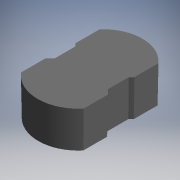
# Autodesk Inventor part: LZ80_Gehaeuse_Parallelform
Saved by Autodesk Inventor 2021 (Build 250183000, 183)
## iProperties
Part Number: LZ80_Gehaeuse_Parallelform
Material: Generic
Catalog Web Link: www.cadenas.de
Description: LZ80 Gehaeuse Parallelform-Bauteil LZ80
Vendor: ROSEKRIEGER
Document SubType Name: Modeling
Designer: partserver
Manufacturer: ROSEKRIEGER
Mass: 1239.51 g
Surface Area: 731.392 cm^2
Volume: 1239.51 cm^3
Density: 1 g/cm^3
Appearance: PSOLRGB-128-128-128
Category: PARTsolutions
Company: ROSEKRIEGER
PSOL_IDENT_0: {$CADENAS_DATA\23d-libs\rose_krieger\linearkomponenten\pool_lineartechnik\_hubsaeule_zyliinder\elekt
PSOL_IDENT_1: rozylinder\elekzyl_lz80\lz80_gehaeuse_parallelform.prj},203 {VTYP=3D},{NB=LZ80_Gehaeuse_Parallelform
PSOL_IDENT_2: },{LINA=LZ80_Gehaeuse_Parallelform},{NN=LZ80 Gehaeuse Parallelform},{DATE=02.12.2020 11:16:40},{GEOM
PSOL_IDENT_3: DATE=12.12.2006},{VERSION=},{LINEID=10},{WBVAR=},{WBNUMERIC=}  {NB=LZ80_Gehaeuse_Parallelform},{LINA=
PSOL_IDENT_4: LZ80_Gehaeuse_Parallelform},{KT=DUMMY},{IDNR=},{ARTIKEL=LZ80_Gehaeuse_Parallelform},{DECKELBR1=107.3
PSOL_IDENT_5: 10},{DECKELBR2=114.310},{DECKELBR3=97.310},{KONTRA1=71.450},{KONTRA2=74.100},{ABKONTRA2=25.250},{ABK
PSOL_IDENT_6: ONTRA1=25.240},{ACHSAB=95.760},{HOEHE=67.000},{ABBEFBO1=56.500},{NUTTIEF=0.100},{NUTBREIT=12.000}
NB: LZ80_Gehaeuse_Parallelform
NN: LZ80 Gehaeuse Parallelform
NT: Bauteil LZ80
NBSYN: $ARTIKEL.
LINA: LZ80_Gehaeuse_Parallelform
CATALOG: RK Rose+Krieger
ARTIKEL: LZ80_Gehaeuse_Parallelform
DECKELBR1: 107.31
DECKELBR2: 114.31
DECKELBR3: 97.31
KONTRA1: 71.45
KONTRA2: 74.1
ABKONTRA2: 25.25
ABKONTRA1: 25.24
ACHSAB: 95.76
HOEHE: 67
ABBEFBO1: 56.5
NUTTIEF: 0.1
NUTBREIT: 12
SUPPLIER: ROSEKRIEGER
ARTICLENO: LZ80_Gehaeuse_Parallelform
BOMINFO: LZ80_Gehaeuse_Parallelform
CREATOR: CADENAS GmbH
Title: LZ80_Gehaeuse_Parallelform
Author: Cadenas PARTsolutions
Comments: Bauteil LZ80
Autodesk Inventor part; units mm, degrees
sketch "Skizze_1" plane through (0, 0, 0) normal (0, 0, 1) x (1, 0, 0)
  line L0 (-57.155, -41.88) -> (-57.055, -41.88)
  line L1 (-57.055, -41.88) -> (-57.055, -53.88)
  line L2 (-57.055, -53.88) -> (-57.155, -53.88)
  line L3 (-57.155, -53.88) -> (-57.155, -69.7905)
  arc A0 (-57.155, -69.7905) -> (57.155, -69.7905) centre (0, -22.63) ccw
  line L4 (57.155, -69.7905) -> (57.155, -53.88)
  line L5 (57.155, -53.88) -> (57.055, -53.88)
  line L6 (57.055, -53.88) -> (57.055, -41.88)
  line L7 (57.055, -41.88) -> (57.155, -41.88)
  line L8 (57.155, -41.88) -> (57.155, -25.9695)
  arc A1 (57.155, -25.9695) -> (48.655, -17.2417) centre (0, -73.13) ccw
  line L9 (48.655, -17.2417) -> (48.655, 20.7961)
  arc A2 (48.655, 20.7961) -> (53.655, 25.9369) centre (0, 73.12) ccw
  line L10 (53.655, 25.9369) -> (53.655, 41.88)
  line L11 (53.655, 41.88) -> (53.555, 41.88)
  line L12 (53.555, 41.88) -> (53.555, 53.88)
  line L13 (53.555, 53.88) -> (53.655, 53.88)
  line L14 (53.655, 53.88) -> (53.655, 69.8231)
  arc A3 (53.655, 69.8231) -> (-53.655, 69.8231) centre (0, 22.64) ccw
  line L15 (-53.655, 69.8231) -> (-53.655, 53.88)
  line L16 (-53.655, 53.88) -> (-53.555, 53.88)
  line L17 (-53.555, 53.88) -> (-53.555, 41.88)
  line L18 (-53.555, 41.88) -> (-53.655, 41.88)
  line L19 (-53.655, 41.88) -> (-53.655, 25.9369)
  arc A4 (-53.655, 25.9369) -> (-48.655, 20.7961) centre (0, 73.12) ccw
  line L20 (-48.655, 20.7961) -> (-48.655, -17.2417)
  arc A5 (-48.655, -17.2417) -> (-57.155, -25.9695) centre (0, -73.13) ccw
  line L21 (-57.155, -25.9695) -> (-57.155, -41.88)
  constraints: 44 end point, 12 point on circle, 6 centre point
extrude "Extrusion1" add sketch "Skizze_1" along normal blind 67 draft -1
ref_plane "EPDOPPELNUT2_XY" through (0, 47.88, 0) normal (0, 0, 1) x (1, 0, 0)
ref_plane "EPDOPPELNUT2_YZ" through (0, 47.88, 0) normal (1, 0, 0) x (0, 1, 0)
ref_plane "EPDOPPELNUT2_ZX" through (0, 47.88, 0) normal (0, 1, 0) x (0, 0, 1)
ref_plane "EPDOPPROFIL_XY" through (0, 47.88, 67) normal (0, 0, 1) x (1, 0, 0)
ref_plane "EPDOPPROFIL_YZ" through (0, 47.88, 67) normal (1, 0, 0) x (0, 1, 0)
ref_plane "EPDOPPROFIL_ZX" through (0, 47.88, 67) normal (0, 1, 0) x (0, 0, 1)
ref_plane "EPFUNKTIONSPR2_XY" through (0, -47.88, 0) normal (0, 0, 1) x (1, 0, 0)
ref_plane "EPFUNKTIONSPR2_YZ" through (0, -47.88, 0) normal (1, 0, 0) x (0, 1, 0)
ref_plane "EPFUNKTIONSPR2_ZX" through (0, -47.88, 0) normal (0, 1, 0) x (0, 0, 1)
ref_plane "EPKONPROFIL_XY" through (0, -47.88, 67) normal (0, 0, 1) x (1, 0, 0)
ref_plane "EPKONPROFIL_YZ" through (0, -47.88, 67) normal (1, 0, 0) x (0, 1, 0)
ref_plane "EPKONPROFIL_ZX" through (0, -47.88, 67) normal (0, 1, 0) x (0, 0, 1)
body "Solid1"
